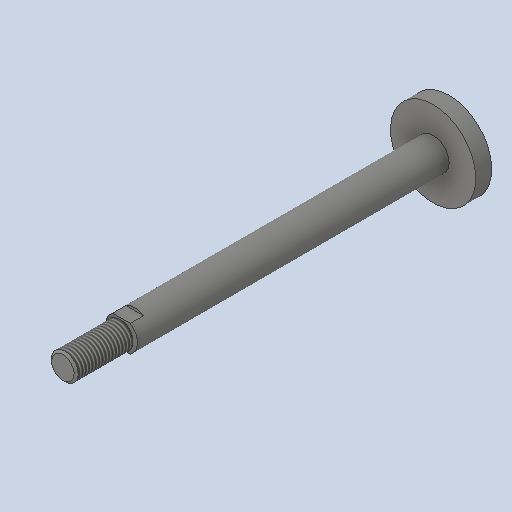
# Autodesk Inventor part: DNC-32-50---(KS)_CPY_CPY
Saved by Autodesk Inventor 2023 (Build 270158000, 158)
## iProperties
Created: 2023-04-07
Part Number: DNC-32-50---(KS)_CPY_CPY
Material: Generic
Catalog Web Link: www.cadenas.de
Description: DNC-(KS)-Standard cylinder
Vendor: FESTO
Document SubType Name: Modeling
Designer: Lenovo
Manufacturer: FESTO
Mass: 19.7253 g
Surface Area: 73.2106 cm^2
Volume: 19.7253 cm^3
Density: 1 g/cm^3
Appearance: PSOLRGB-128-128-128
Category: PARTsolutions
Company: FESTO
Title: DNC-32-50---(KS)
Author: Cadenas PARTsolutions
Comments: Standard cylinder
PSOL_IDENT_0: {$CADENAS_DATA/23d-libs/festo/parts/d/dnc/parts/dnc_kst.prj},232 {VTYP=3D},{NB=DNC-32-50---(KS)},{LI
PSOL_IDENT_1: NA=DNC-32-50---(KS)},{NN=DNC-(KS)},{DATE=06.03.2020 08:57:36},{GEOMDATE=06.03.2020 08:57:36},{VERSIO
PSOL_IDENT_2: N=},{LINEID=10},{WBVAR=HUB,KP,Q,S2,K2,K3,K5,K7,K8,TT},{WBNUMERIC=HUB,KP,Q,S2,K2,K3,K5,K7,K8,TT}  {NB=
PSOL_IDENT_3: DNC-32-50---(KS)},{LINA=DNC-32-50---(KS)},{KT=DUMMY},{TNR=},{TYP=DNC},{KDM=32},{MASSBASIC=0.162},{MA
PSOL_IDENT_4: SSHUB=0.009},{HUB=50},{KP=0},{Q=0},{S2=1},{K2=0},{K3=0},{K5=0},{K7=0},{K8=0},{TT=0},{ZZ=0.1},{AM=22.
PSOL_IDENT_5: 000},{A1=35.000},{A2=500.000},{B=30.000},{B1=10.000},{D1=M6},{D1N=6.000},{D1K=4.917},{D2=12.000},{D8=
PSOL_IDENT_6: 4.5},{KK=M10x1,25},{KKN=10.000},{KKP=1.250},{KKK=8.160},{K1=M10},{K1N=10.000},{K1K=8.160},{L4=4.000}
PSOL_IDENT_7: ,{L5=25.100},{L8=10.000},{L15=148.000},{SW2=10.000},{T=12.000},{VD=18.000},{WH=26.000},{ZB=120.000},
PSOL_IDENT_8: {X=2.600},{KPT=},{KPN=0},{QT=},{QN=0},{S2T=},{S2N=1},{K2T=},{K3N=0},{K3T=},{K5N=0},{K5T=},{K7N=0},{K
PSOL_IDENT_9: 7T=},{K8T=},{TTT=},{LKP=45.000},{ZM=123},{KPMONT=0},{LKPAD=0},{LKPLD=0},{L15K=2},{XF31=4.000},{B31=5
PSOL_IDENT_10: .000},{V1=1.000}
NB: DNC-32-50---(KS)
NN: DNC-(KS)
NT: Standard cylinder
NBSYN: $TYP.-$KDM.-$HUB.$KPT.$QT.$S2T.$K2T.$K3T.$K5T.$K7T.$K8T.$TTT.---(KS)
LINA: DNC-32-50---(KS)
CATALOG: Festo
TYP: DNC
KDM: 32
MASSBASIC: 0.162
MASSHUB: 0.009
HUB: 50
KP: ohne
Q: rund
S2: 1
K2: 0
K3: Aussengewinde
K5: standard
K7: standard
K8: 0
TT: -
AM: 22
A1: 35
A2: 500
B: 30
B1: 10
D1: M6
D1N: 6
D1K: 4.917
D2: 12
D8: 4.5
KK: M10x1,25
KKN: 10
KKP: 1.25
KKK: 8.16
K1: M10
K1N: 10
K1K: 8.16
L4: 4
L5: 25.1
L8: 10
L15: 148
SW2: 10
T: 12
VD: 18
WH: 26
ZB: 120
X: 2.6
LKP: 45
L15K: 2
XF31: 4
B31: 5
V1: 1
SUPPLIER: FESTO
ARTICLENO: DNC-32-50---(KS)
BOMINFO: DNC-32-50---(KS)
CREATOR: CADENAS GmbH
Autodesk Inventor part; units mm, degrees
sketch "Base_KS" plane through (0, 0, 0) normal (1, 0, 0) x (0, 1, 0)
  line L0 (0, 0) -> (0, 122.9)
  line L1 (0, 122.9) -> (3, 122.9)
  line L2 (3, 122.9) -> (3, 6)
  line L3 (3, 6) -> (16, 6)
  line L4 (16, 6) -> (16, 0)
  line L5 (16, 0) -> (0, 0)
  line L6 (0, 0) -> (0, 122.9)
  constraints: 14 end point
revolve "Revolution1" add sketch "Base_KS" angle 360 about axis through (0, 0, 0) along (0, 0, -1)
sketch "Skizze_2" plane through (0, 0, 0) normal (1, 0, 0) x (0, 1, 0)
  line L0 (0, 0.1) -> (0, 123)
  line L1 (0, 123) -> (6, 123)
  line L2 (6, 123) -> (6, 0.1)
  line L3 (6, 0.1) -> (0, 0.1)
  line L4 (0, 0.1) -> (0, 123)
  constraints: 10 end point
revolve "Revolution2" add sketch "Skizze_2" angle 360 about axis through (0, 0, 0.1) along (0, 0, -1)
sketch "Skizze_4" plane through (0, 0, 123) normal (0, 0, 1) x (0, 1, 0)
  line L0 (5, 12) -> (5, -12)
  line L1 (5, -12) -> (12, -12)
  line L2 (12, -12) -> (12, 12)
  line L3 (12, 12) -> (5, 12)
  constraints: 8 end point
extrude "Extrusion1" cut sketch "Skizze_4" along normal mid plane 10
sketch "Skizze_5" plane through (0, 0, 123) normal (0, 0, 1) x (0, 1, 0)
  line L0 (-12, 12) -> (-12, -12)
  line L1 (-12, -12) -> (-5, -12)
  line L2 (-5, -12) -> (-5, 12)
  line L3 (-5, 12) -> (-12, 12)
  constraints: 8 end point
extrude "Extrusion2" cut sketch "Skizze_5" along normal mid plane 10
sketch "Skizze_8" plane through (0, 0, 0) normal (1, 0, 0) x (0, 1, 0)
  line L0 (0, 122.9) -> (0, 145)
  line L1 (0, 145) -> (4.233, 145)
  line L2 (4.233, 145) -> (5, 144.233)
  line L3 (5, 144.233) -> (5, 123.667)
  line L4 (5, 123.667) -> (4.233, 122.9)
  line L5 (4.233, 122.9) -> (0, 122.9)
  line L6 (0, 122.9) -> (0, 145)
  constraints: 14 end point
revolve "Revolution3" add sketch "Skizze_8" angle 360 about axis through (0, 0, 122.9) along (0, 0, -1)
thread "Thread1" size "M10x1.25" class "6g" standard "ISO Metric profile" full length
ref_plane "ANSCHRAUB_XY" through (0, 0, 145) normal (0, 0, 1) x (1, 0, 0)
ref_plane "ANSCHRAUB_YZ" through (0, 0, 145) normal (1, 0, 0) x (0, 1, 0)
ref_plane "ANSCHRAUB_ZX" through (0, 0, 145) normal (0, 1, 0) x (0, 0, 1)
ref_plane "CP_30_XY" through (0, 0, 123) normal (0, 0, 1) x (1, 0, 0)
ref_plane "CP_30_YZ" through (0, 0, 123) normal (1, 0, 0) x (0, 1, 0)
ref_plane "CP_30_ZX" through (0, 0, 123) normal (0, 1, 0) x (0, 0, 1)
ref_plane "KS_AUFSATZ1_XY" through (0, 0, 132) normal (0, 0, 1) x (1, 0, 0)
ref_plane "KS_AUFSATZ1_YZ" through (0, 0, 132) normal (1, 0, 0) x (0, 1, 0)
ref_plane "KS_AUFSATZ1_ZX" through (0, 0, 132) normal (0, 1, 0) x (0, 0, 1)
ref_plane "NUT1_XY" through (0, 0, 132) normal (0, 0, -1) x (1, 0, 0)
ref_plane "NUT1_YZ" through (0, 0, 132) normal (1, 0, 0) x (0, -1, 0)
ref_plane "NUT1_ZX" through (0, 0, 132) normal (0, -1, 0) x (0, 0, -1)
ref_plane "ZYLINDER_XY" through (0, 0, 0) normal (0, 0, 1) x (1, 0, 0)
ref_plane "ZYLINDER_YZ" through (0, 0, 0) normal (1, 0, 0) x (0, 1, 0)
ref_plane "ZYLINDER_ZX" through (0, 0, 0) normal (0, 1, 0) x (0, 0, 1)
body "Solid1"
